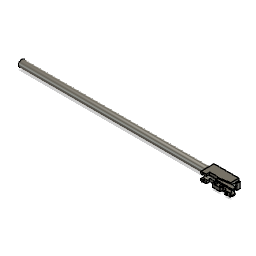
LP-point V2 (Autodesk Fusion 360 archive; units mm, degrees)
design "hp-995 barrel"
Autodesk Fusion 360 part; units mm, degrees
sketch "Sketch1" plane through (0, 0, 0) normal (0, 1, 0) x (1, 0, 0)
  line L0 (0, 0) -> (59, -0.000123)
  line L1 (0, 0) -> (59, -0.000123)
  line L2 (59, -0.000123) -> (58.999962, -18.000123)
  line L3 (0, 0) -> (-0.000063, -30)
  line L4 (-0.000063, -30) -> (4.999937, -30.00001)
  line L5 (4.999937, -30.00001) -> (4.999937, -29.00001)
  line L6 (4.999937, -29.000011) -> (11.499972, -29.000024)
  line L7 (11.499972, -29.000024) -> (11.499989, -21.000024)
  line L8 (11.499989, -21.000024) -> (30.499989, -21.000064)
  line L9 (30.49999, -21.000064) -> (30.499961, -34.49993)
  line L10 (59, -0.000123) -> (59, -11)
  line L11 (59, -0.000123) -> (58.999962, -18.000123)
  line L12 (58.999962, -18.000123) -> (64.000056, -18.000122)
  line L13 (68.499973, -21.000073) -> (68.499955, -30.000009)
  line L14 (68.499973, -21.000073) -> (64.000056, -18.000122)
  line L15 (68.499973, -21.000073) -> (68.499964, -25.500073)
  line L16 (70.000004, -33.000003) -> (70.000008, -31.000046)
  line L17 (0, 0) -> (59, -0.000123)
  line L18 (70.000008, -31.000046) -> (70.000004, -33.000003)
  line L19 (68.499955, -30.000009) -> (70.000008, -31.000046)
  line L20 (69.499995, -33.500012) -> (70.000004, -33.000003)
  line L21 (70, -35.000046) -> (70.000001, -34.5)
  circle A0 centre (34.5, -29.5) radius 2.5
  circle A1 centre (45.5, -29.5) radius 2.5
  line L22 (30.499961, -34.49993) -> (47.998896, -34.499967)
  line L23 (58.998896, -34.49999) -> (63.932836, -34.5)
  line L24 (50.387631, -29.964548) -> (56.610162, -29.964548)
  arc A2 (58.998896, -34.49999) -> (56.610162, -29.964548) centre (53.498896, -34.499967) ccw
  arc A3 (50.387631, -29.964548) -> (47.998896, -34.499967) centre (53.498896, -34.499967) ccw
  line L25 (63.932836, -34.5) -> (63.932838, -33.5)
  line L26 (63.932838, -33.5) -> (69.499995, -33.500012)
  dimension "d3" = 59
  dimension "d7" = 30
  dimension "d8" = 5
  dimension "d9" = 1
  dimension "d11" = 8
  dimension "d12" = 19
  dimension "d19" = 18
  dimension "d24" = 4.5
  dimension "d27" = 4
  dimension "d34" = 5.5
  dimension "d36" = 1
  constraint coincident L0.start L1.start
  constraint perpendicular L0 L2
  constraint perpendicular L1 L3
  constraint perpendicular L3 L4
  constraint vertical L5
  constraint perpendicular L3 L6
  constraint perpendicular L6 L7
  constraint perpendicular L7 L8
  constraint perpendicular L1 L9
  constraint perpendicular L0 L11
  constraint perpendicular L9 L22
  constraint parallel L13 L15
  constraint perpendicular L3 L17
  constraint perpendicular L17 L18
  constraint parallel L3 L13
  constraint collinear L22 L23
  constraint horizontal L24
  constraint concentric A2 A3
  constraint perpendicular L23 L25
  constraint perpendicular L25 L26
extrude "Extrude1" add sketch "Sketch1" along normal blind 18.5 contours L0 L1 L2 L3 L4 L5 L6 L7 L8 L9 L10 L11 L12 L13 L14 L15 L16 L17 L18 L19 L20 L22 L23 L24 A2 A3 L25 L26 picked at (29.83333, -7.000062) makes body 1
sketch "Sketch2" plane through (0, 0, 0) normal (1, 0, 0) x (0, 0, -1)
  line L0 (0, 0) -> (0, 18.5)
  line L1 (-19, 9.25) -> (-19, 9.252074)
  circle A0 centre (-11.4, 9.25) radius 7.6
  dimension "d39" = 18.5
  constraint coincident L0.start origin
  constraint vertical L0
  measures "d39" distance of L0.start L0.end
extrude "Extrude2" add sketch "Sketch2" against normal blind 422 contours L1 A0 picked at (-8.894962, 8.872426) bodies 1
sketch "Sketch3" plane through (0, 0, 0) normal (0, 1, 0) x (1, 0, 0)
sketch "Sketch4" plane through (0, 18.5, 0) normal (0, 1, 0) x (-1, 0, 0)
  circle A0 centre (-34.5, 29.5) radius 2.5
  circle A1 centre (-45.5, 29.5) radius 2.5
  line L0 (-58.998896, 34.49999) -> (-63.932836, 34.5)
  line L1 (-63.932836, 34.5) -> (-63.932838, 33.5)
  line L2 (-63.932838, 33.5) -> (-69.499995, 33.500012)
  line L3 (-69.499995, 33.500012) -> (-70.000004, 33.000003)
  line L4 (-70.000004, 33.000003) -> (-70.000008, 31.000046)
  line L5 (-70.000008, 31.000046) -> (-68.499955, 30.000009)
  line L6 (-68.499955, 30.000009) -> (-68.499973, 21.000073)
  line L7 (-68.499973, 21.000073) -> (-64.000056, 18.000122)
  line L8 (-64.000056, 18.000122) -> (-58.999962, 18.000123)
  line L9 (-58.999962, 18.000123) -> (-59, 0.000123)
  line L10 (-59, 0.000123) -> (0, 0)
  line L11 (0, 0) -> (0.000063, 30)
  line L12 (0.000063, 30) -> (-4.999937, 30.00001)
  line L13 (-4.999937, 30.00001) -> (-4.999937, 29.000011)
  line L14 (-4.999937, 29.000011) -> (-11.499972, 29.000024)
  line L15 (-11.499972, 29.000024) -> (-11.499989, 21.000024)
  line L16 (-11.499989, 21.000024) -> (-30.49999, 21.000064)
  line L17 (-30.49999, 21.000064) -> (-30.499961, 34.49993)
  line L18 (-30.499961, 34.49993) -> (-47.998896, 34.499967)
  arc A2 (-50.387631, 29.964548) -> (-47.998896, 34.499967) centre (-53.498896, 34.499967) ccw
  line L19 (-50.387631, 29.964548) -> (-56.610162, 29.964548)
  arc A3 (-58.998896, 34.49999) -> (-56.610162, 29.964548) centre (-53.498896, 34.499967) ccw
  line L20 (-58.999962, 18.000123) -> (-55.999962, 18.000117)
  line L21 (-55.999962, 18.000117) -> (-56, 0.000117)
  line L22 (-58.999962, 18.000123) -> (-59, 0.000123)
  line L23 (-59, 0.000123) -> (-56, 0.000117)
  dimension "d44" = 3
  constraint perpendicular L9 L20
  constraint perpendicular L10 L21
extrude "Extrude3" cut sketch "Sketch4" against normal blind 5 contours L9 L10 L20 L21 L22 L23 picked at (-57.999987, 6.000121) bodies 1
sketch "Sketch5" plane through (-422, 0, 0) normal (-1, 0, 0) x (0, 0, 1)
  circle A0 centre (11.4, 9.25) radius 7.6
  circle A1 centre (11.4, 9.25) radius 4.5
  dimension "d47" = 9
  constraint concentric A0 A1
  measures "d47" diameter of A1
extrude "Extrude4" cut sketch "Sketch5" against normal blind 500 contours A1 picked at (10.485657, 10.143968) bodies 1
sketch "Sketch6" plane through (0, 0, 0) normal (-1, 0, -0.00000209) x (-0.00000209, 0, 1)
  ellipse E0 centre (11.4, 9.25) end of major axis (3.8, 9.25) minor radius 7.6
  line L0 (0, 0) -> (30, 0)
  line L1 (30, 0) -> (30, 18.5)
  line L2 (30, 18.5) -> (0, 18.5)
  line L3 (0, 18.5) -> (0, 0)
  line L4 (30, 18.5) -> (30, 0)
  line L5 (25.100054, 14.248999) -> (30, 14.150928)
  line L6 (25.100054, 4.251001) -> (30, 4.349072)
  arc A0 (25.100054, 14.248999) -> (25.100054, 4.251001) centre (25, 9.25) ccw
  constraint coincident L1.end L2.start
  constraint coincident L0 L1.start
  constraint coincident L1 L0.end
  constraint tangent L5 A0
  constraint tangent L6 A0
extrude "Extrude5" cut sketch "Sketch6" against normal blind 29 contours L1 L4 L5 L6 A0 picked at (26.733369, 10.883643) bodies 1
sketch "Sketch7" plane through (0, 18.5, 0) normal (0, 1, 0) x (-1, 0, 0)
  line L0 (-55.999962, 18.000117) -> (-56, 0.000117)
  line L1 (-56, 0.000117) -> (0, 0)
  line L2 (0, 0) -> (0.000063, 30)
  line L3 (0.000063, 30) -> (-4.999937, 30.00001)
  line L4 (-4.999937, 30.00001) -> (-4.999937, 29.000011)
  line L5 (-4.999937, 29.000011) -> (-11.499972, 29.000024)
  line L6 (-11.499972, 29.000024) -> (-11.499989, 21.000024)
  line L7 (-11.499989, 21.000024) -> (-30.49999, 21.000064)
  line L8 (-30.49999, 21.000064) -> (-30.499961, 34.49993)
  line L9 (-30.499961, 34.49993) -> (-47.998896, 34.499967)
  arc A0 (-50.387631, 29.964548) -> (-47.998896, 34.499967) centre (-53.498896, 34.499967) ccw
  line L10 (-50.387631, 29.964548) -> (-56.610162, 29.964548)
  arc A1 (-58.998896, 34.49999) -> (-56.610162, 29.964548) centre (-53.498896, 34.499967) ccw
  line L11 (-58.998896, 34.49999) -> (-63.932836, 34.5)
  line L12 (-63.932836, 34.5) -> (-63.932838, 33.5)
  line L13 (-63.932838, 33.5) -> (-69.499995, 33.500012)
  line L14 (-69.499995, 33.500012) -> (-70.000004, 33.000003)
  line L15 (-70.000004, 33.000003) -> (-70.000008, 31.000046)
  line L16 (-70.000008, 31.000046) -> (-68.499955, 30.000009)
  line L17 (-68.499955, 30.000009) -> (-68.499973, 21.000073)
  line L18 (-68.499973, 21.000073) -> (-64.000056, 18.000122)
  line L19 (-64.000056, 18.000122) -> (-58.999962, 18.000123)
  line L20 (-58.999962, 18.000123) -> (-55.999962, 18.000117)
  circle A2 centre (-34.5, 29.5) radius 2.5
  circle A3 centre (-45.5, 29.5) radius 2.5
  line L21 (-30.499961, 34.49993) -> (-30.499978, 26.49993)
  line L22 (-30.499978, 26.49993) -> (-68.499962, 26.50001)
  dimension "d53" = 8
  constraint perpendicular L9 L21
  constraint perpendicular L17 L22
extrude "Extrude6" cut sketch "Sketch7" against normal blind 5.5 contours L8 L9 A0 L10 A1 L11 L12 L13 L14 L15 L16 L17 L21 L22 picked at (-63.388235, 30.329444) bodies 1
sketch "Sketch8" plane through (0, 0, 0) normal (0, -1, 0) x (1, 0, 0)
  circle A0 centre (34.5, 29.5) radius 2.5
  circle A1 centre (45.5, 29.5) radius 2.5
  line L0 (63.932836, 34.5) -> (58.998896, 34.49999)
  arc A2 (56.610162, 29.964548) -> (58.998896, 34.49999) centre (53.498896, 34.499967) ccw
  line L1 (56.610162, 29.964548) -> (50.387631, 29.964548)
  arc A3 (47.998896, 34.499967) -> (50.387631, 29.964548) centre (53.498896, 34.499967) ccw
  line L2 (47.998896, 34.499967) -> (30.499961, 34.49993)
  line L3 (30.499961, 34.49993) -> (30.49999, 21.000064)
  line L4 (30.49999, 21.000064) -> (11.499989, 21.000024)
  line L5 (11.499989, 21.000024) -> (11.499972, 29.000024)
  line L6 (11.499972, 29.000024) -> (4.999937, 29.000011)
  line L7 (4.999937, 29.000011) -> (4.999937, 30.00001)
  line L8 (4.999937, 30.00001) -> (-0.000063, 30)
  line L9 (-0.000063, 30) -> (0, 0)
  line L10 (0, 0) -> (59, 0.000123)
  line L11 (59, 0.000123) -> (58.999962, 18.000123)
  line L12 (58.999962, 18.000123) -> (64.000056, 18.000122)
  line L13 (64.000056, 18.000122) -> (68.499973, 21.000073)
  line L14 (68.499973, 21.000073) -> (68.499955, 30.000009)
  line L15 (68.499955, 30.000009) -> (70.000008, 31.000046)
  line L16 (70.000008, 31.000046) -> (70.000004, 33.000003)
  line L17 (70.000004, 33.000003) -> (69.499995, 33.500012)
  line L18 (69.499995, 33.500012) -> (63.932838, 33.5)
  line L19 (63.932838, 33.5) -> (63.932836, 34.5)
  line L20 (30.499961, 34.49993) -> (30.499978, 26.49993)
  line L21 (30.499978, 26.49993) -> (68.499962, 26.50001)
  dimension "d56" = 8
  constraint perpendicular L2 L20
  constraint perpendicular L14 L21
extrude "Extrude7" cut sketch "Sketch8" against normal blind 5.5 contours L0 A2 L1 A3 L2 L3 L14 L15 L16 L17 L18 L19 L20 L21 picked at (63.388235, 30.329444) bodies 1
sketch "Sketch9" plane through (0, 0, 0) normal (0, -1, 0) x (1, 0, 0)
  line L0 (68.499962, 26.50001) -> (30.499978, 26.49993)
  line L1 (30.499978, 26.49993) -> (30.49999, 21.000064)
  line L2 (30.49999, 21.000064) -> (11.499989, 21.000024)
  line L3 (11.499989, 21.000024) -> (11.499972, 29.000024)
  line L4 (11.499972, 29.000024) -> (4.999937, 29.000011)
  line L5 (4.999937, 29.000011) -> (4.999937, 30.00001)
  line L6 (4.999937, 30.00001) -> (-0.000063, 30)
  line L7 (-0.000063, 30) -> (0, 0)
  line L8 (0, 0) -> (59, 0.000123)
  line L9 (59, 0.000123) -> (58.999962, 18.000123)
  line L10 (58.999962, 18.000123) -> (64.000056, 18.000122)
  line L11 (64.000056, 18.000122) -> (68.499973, 21.000073)
  line L12 (68.499973, 21.000073) -> (68.499962, 26.50001)
  line L13 (30.499978, 26.49993) -> (30.499986, 22.49993)
  line L14 (30.499986, 22.49993) -> (68.49997, 22.50001)
  dimension "d59" = 4
  constraint perpendicular L0 L13
  constraint perpendicular L12 L14
extrude "Extrude8" cut sketch "Sketch9" against normal blind 2.5 contours L0 L1 L12 L13 L14 picked at (43.166642, 25.166623) bodies 1
sketch "Sketch10" plane through (0, 18.5, 0) normal (0, 1, 0) x (-1, 0, 0)
  line L0 (-30.499978, 26.49993) -> (-68.499962, 26.50001)
  line L1 (-68.499962, 26.50001) -> (-68.499973, 21.000073)
  line L2 (-68.499973, 21.000073) -> (-64.000056, 18.000122)
  line L3 (-64.000056, 18.000122) -> (-58.999962, 18.000123)
  line L4 (-58.999962, 18.000123) -> (-55.999962, 18.000117)
  line L5 (-55.999962, 18.000117) -> (-56, 0.000117)
  line L6 (-56, 0.000117) -> (0, 0)
  line L7 (0, 0) -> (0.000063, 30)
  line L8 (0.000063, 30) -> (-4.999937, 30.00001)
  line L9 (-4.999937, 30.00001) -> (-4.999937, 29.000011)
  line L10 (-4.999937, 29.000011) -> (-11.499972, 29.000024)
  line L11 (-11.499972, 29.000024) -> (-11.499989, 21.000024)
  line L12 (-11.499989, 21.000024) -> (-30.49999, 21.000064)
  line L13 (-30.49999, 21.000064) -> (-30.499978, 26.49993)
  line L14 (-30.499978, 26.49993) -> (-30.499986, 22.49993)
  line L15 (-30.499986, 22.49993) -> (-68.49997, 22.50001)
  dimension "d62" = 4
  constraint perpendicular L12 L14
  constraint perpendicular L1 L15
extrude "Extrude9" cut sketch "Sketch10" against normal blind 2.5 contours L0 L1 L13 L14 L15 picked at (-43.166642, 25.166623) bodies 1
sketch "Sketch11" plane through (0, 18.5, 0) normal (0, 1, 0) x (-1, 0, 0)
  line L0 (-30.499986, 22.49993) -> (-68.49997, 22.50001)
  line L1 (-68.49997, 22.50001) -> (-68.499973, 21.000073)
  line L2 (-68.499973, 21.000073) -> (-64.000056, 18.000122)
  line L3 (-64.000056, 18.000122) -> (-58.999962, 18.000123)
  line L4 (-58.999962, 18.000123) -> (-55.999962, 18.000117)
  line L5 (-55.999962, 18.000117) -> (-56, 0.000117)
  line L6 (-56, 0.000117) -> (0, 0)
  line L7 (0, 0) -> (0.000063, 30)
  line L8 (0.000063, 30) -> (-4.999937, 30.00001)
  line L9 (-4.999937, 30.00001) -> (-4.999937, 29.000011)
  line L10 (-4.999937, 29.000011) -> (-11.499972, 29.000024)
  line L11 (-11.499972, 29.000024) -> (-11.499989, 21.000024)
  line L12 (-11.499989, 21.000024) -> (-30.49999, 21.000064)
  line L13 (-30.49999, 21.000064) -> (-30.499986, 22.49993)
  line L14 (-30.499986, 22.49993) -> (-55.999962, 18.000117)
extrude "Extrude10" cut sketch "Sketch11" against normal blind 2.5 contours L0 L1 L2 L3 L4 L14 picked at (-51.66664, 21.000019) bodies 1
sketch "Sketch12" plane through (0, 0, 0) normal (0, -1, 0) x (1, 0, 0)
  line L0 (68.49997, 22.50001) -> (30.499986, 22.49993)
  line L1 (30.499986, 22.49993) -> (30.49999, 21.000064)
  line L2 (30.49999, 21.000064) -> (11.499989, 21.000024)
  line L3 (11.499989, 21.000024) -> (11.499972, 29.000024)
  line L4 (11.499972, 29.000024) -> (4.999937, 29.000011)
  line L5 (4.999937, 29.000011) -> (4.999937, 30.00001)
  line L6 (4.999937, 30.00001) -> (-0.000063, 30)
  line L7 (-0.000063, 30) -> (0, 0)
  line L8 (0, 0) -> (59, 0.000123)
  line L9 (59, 0.000123) -> (58.999962, 18.000123)
  line L10 (58.999962, 18.000123) -> (64.000056, 18.000122)
  line L11 (64.000056, 18.000122) -> (68.499973, 21.000073)
  line L12 (68.499973, 21.000073) -> (68.49997, 22.50001)
  line L13 (58.999962, 18.000123) -> (30.499986, 22.49993)
extrude "Extrude11" cut sketch "Sketch12" against normal blind 2.5 contours L0 L10 L11 L12 L13 picked at (52.66664, 21.000021) bodies 1
sketch "Sketch13" plane through (-0.000072, 0, 34.499867) normal (-0.00000209, 0, 1) x (1, 0, 0.00000209)
  line L0 (58.998968, 5.5) -> (63.932908, 5.5)
  line L1 (63.932908, 5.5) -> (63.932908, 13)
  line L2 (63.932908, 13) -> (58.998968, 13)
  line L3 (58.998968, 13) -> (58.998968, 5.5)
  circle A0 centre (61.465938, 9.25) radius 1.5
  dimension "d69" = 3
  measures "d69" diameter of A0
extrude "Extrude12" add sketch "Sketch13" along normal blind 1 contours A0 picked at (61.81025, 9.442709) bodies 1
sketch "Sketch14" plane through (0, 0, 0) normal (0, -1, 0) x (1, 0, 0)
  line L0 (58.999962, 18.000123) -> (30.499986, 22.49993)
  line L1 (30.499986, 22.49993) -> (30.49999, 21.000064)
  line L2 (30.49999, 21.000064) -> (11.499989, 21.000024)
  line L3 (11.499989, 21.000024) -> (11.499972, 29.000024)
  line L4 (11.499972, 29.000024) -> (4.999937, 29.000011)
  line L5 (4.999937, 29.000011) -> (4.999937, 30.00001)
  line L6 (4.999937, 30.00001) -> (-0.000063, 30)
  line L7 (-0.000063, 30) -> (0, 0)
  line L8 (0, 0) -> (59, 0.000123)
  line L9 (59, 0.000123) -> (58.999962, 18.000123)
  line L10 (59, 0.000123) -> (58.999984, 7.500123)
  line L11 (58.999984, 7.500123) -> (55.999984, 7.500117)
  line L12 (55.999972, 13.500117) -> (58.999972, 13.500123)
  line L13 (58.999984, 7.500123) -> (55.999984, 7.500117)
  line L14 (55.999984, 7.500117) -> (55.999972, 13.500117)
  dimension "d72" = 7.5
  dimension "d75" = 3
  constraint perpendicular L8 L10
  constraint perpendicular L9 L11
  constraint perpendicular L9 L12
  constraint perpendicular L9 L13
  constraint perpendicular L12 L14
extrude "Extrude13" cut sketch "Sketch14" against normal blind 20 contours L9 L11 L12 L13 L14 picked at (56.99998, 9.500119) bodies 1
sketch "Sketch15" plane through (59, 0, 0.000123) normal (1, 0, 0.00000209) x (0.00000209, 0, -1)
  line L0 (-13.5, 0) -> (-13.5, 5.270115)
  arc A0 (-13.5, 13.229885) -> (-13.5, 5.270115) centre (-11.399877, 9.25) ccw
  line L1 (-13.5, 13.229885) -> (-13.5, 13.5)
  line L2 (-13.5, 13.5) -> (-18, 13.5)
  line L3 (-18, 13.5) -> (-18, 2.5)
  line L4 (-18, 2.5) -> (-18, 0)
  line L5 (-18, 0) -> (-13.5, 0)
sketch "Sketch16" plane through (51.500017, 0, 51.499997) normal (0.70710691, 0, 0.70710665) x (0.70710665, 0, -0.70710691)
  line L0 (25.455819, 5.5) -> (26.162938, 5.5)
  line L1 (26.162938, 5.5) -> (26.162938, 13)
  line L2 (26.162938, 13) -> (25.455819, 13)
  line L3 (25.455819, 13) -> (25.455819, 5.5)
  line L4 (25.455819, 9.25) -> (26.162938, 9.25)
  line L5 (26.162938, 9.25) -> (30.662938, 9.25)
  circle A0 centre (30.662938, 9.25) radius 4.5
  dimension "d79" = 9
  constraint perpendicular L1 L5
  measures "d79" diameter of A0
extrude "Extrude14" cut sketch "Sketch16" against normal blind 25 contours A0 picked at (32.430079, 10.270259) bodies 1 makes body 2 at (58.974168, 13.499091, 13.51487)

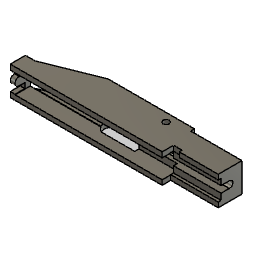
design "995 bolt"
Autodesk Fusion 360 part; units mm, degrees
sketch "Sketch1" plane through (0, 0, 0) normal (0, 1, 0) x (1, 0, 0)
  line L0 (65, 0) -> (156, 0)
  line L1 (0, -22) -> (0, -38)
  line L2 (210, -4) -> (210, -29)
  line L3 (160, -38) -> (0, -38)
  line L4 (156, 0) -> (156, -4)
  line L5 (156, -4) -> (210, -4)
  line L6 (0, -38) -> (0, -22)
  line L7 (0, -22) -> (10, -22)
  line L8 (10, -22) -> (65, 0)
  line L9 (210, 0) -> (135, 0)
  circle A0 centre (135, -8.75) radius 3.25
  line L10 (160, -38) -> (160, -29)
  line L11 (160, -29) -> (210, -29)
  dimension "d2" = 38
  dimension "d5" = 4
  dimension "d6" = 16
  dimension "d7" = 10
  dimension "d8" = 65
  dimension "d9" = 75
  dimension "d13" = 9
  constraint horizontal L0
  constraint perpendicular L0 L1
  constraint perpendicular L0 L2
  constraint perpendicular L0 L4
  constraint perpendicular L4 L5
  constraint perpendicular L3 L6
  constraint perpendicular L1 L7
  constraint parallel L0 L9
  constraint perpendicular L3 L10
  constraint perpendicular L10 L11
  measures "d2" distance of origin L1.end
  measures "d5" distance of L0.end L4.end
  measures "d6" distance of L1.end L1.start
  measures "d7" distance of L1.start L7.end
  measures "d8" distance of origin L0.start
  measures "d9" distance of L9.start L9.end
  measures "d13" distance of L3.start L10.end
extrude "Extrude1" add sketch "Sketch1" along normal blind 30.5
sketch "Sketch2" plane through (0, 30.5, 0) normal (0, 1, 0) x (-1, 0, 0)
  circle A0 centre (-135, 8.75) radius 3.25
  line L0 (-160, 38) -> (-160, 29)
  line L1 (-160, 29) -> (-210, 29)
  line L2 (-210, 29) -> (-210, 4)
  line L3 (-210, 4) -> (-156, 4)
  line L4 (-156, 4) -> (-156, 0)
  line L5 (-156, 0) -> (-65, 0)
  line L6 (-65, 0) -> (-10, 22)
  line L7 (-10, 22) -> (0, 22)
  line L8 (0, 22) -> (0, 38)
  line L9 (0, 38) -> (-160, 38)
  line L10 (-160, 29) -> (-160, 26)
  line L11 (-160, 26) -> (-169, 26)
  line L12 (-169, 26) -> (-169, 29)
  dimension "d16" = 3
  dimension "d17" = 9
  constraint coincident L0.end L1.start
  constraint perpendicular L1 L10
  constraint perpendicular L10 L11
  constraint coincident L1 L12.end
  constraint perpendicular L1 L12
  measures "d16" distance of L0.end L10.end
  measures "d17" distance of L10.end L11.end
extrude "Extrude2" cut sketch "Sketch2" against normal blind 5.5 contours L1 L10 L11 L12
sketch "Sketch3" plane through (0, 0, 0) normal (-1, 0, 0) x (0, 0, 1)
  line L0 (22, 0) -> (38, 0)
  line L1 (38, 0) -> (38, 30.5)
  line L2 (38, 30.5) -> (22, 30.5)
  line L3 (22, 30.5) -> (22, 0)
  line L4 (22, 15.25) -> (38, 15.25)
  line L5 (38, 15.25) -> (33.75, 15.25)
  line L6 (22, 30.5) -> (27.5, 30.5)
  line L7 (33.75, 11) -> (27.5, 11)
  line L8 (33.9717, 19.4942) -> (27.5, 19.4942)
  arc A0 (33.75, 11) -> (33.5283, 19.4942) centre (33.75, 15.25) ccw
  line L9 (27.5, 30.5) -> (27.5, 19.4942)
  line L10 (27.5, 11) -> (27.5, 0)
  line L11 (33.9717, 24.9942) -> (27.5, 24.9942)
  line L12 (33.75, 5.5) -> (27.5, 5.5)
  line L13 (33.75, 5.5) -> (38, 5.5)
  line L14 (33.9717, 24.9942) -> (38, 24.9942)
  dimension "d20" = 4.25
  dimension "d21" = 5.5
  dimension "d22" = 5.5
  dimension "d23" = -5.5
  constraint midpoint L3 L4.start
  constraint midpoint L1 L4.end
  constraint parallel L4 L5
  constraint coincident L5.end A0.centre
  constraint coincident L4.end A0
  constraint coincident L2.end L3.start
  constraint perpendicular L3 L6
  constraint perpendicular L6 L9
  constraint coincident L7.end L9
  constraint tangent L7 A0
  constraint perpendicular L7 L9
  constraint coincident L8.start A0
  constraint perpendicular L8 L9
  constraint coincident L8 A0.end
  constraint collinear L9 L10
  constraint coincident L1 L13.end
  constraint perpendicular L1 L13
  constraint coincident L1 L14.end
  constraint perpendicular L1 L14
  measures "d20" distance of L4.end L5.end
  measures "d21" distance of L2.end L6.end
extrude "Extrude3" cut sketch "Sketch3" against normal blind 300 contours L1 L7 A0 L10 L12 L13 | L1 L8 A0 L9 L11 L14
sketch "Sketch4" plane through (0, 0, 38) normal (0, 0, 1) x (1, 0, 0)
  line L0 (0, 24.9942) -> (160, 24.9942)
  line L1 (160, 24.9942) -> (160, 30.5)
  line L2 (160, 30.5) -> (0, 30.5)
  line L3 (0, 30.5) -> (0, 24.9942)
  line L4 (0, 19) -> (0, 11)
  line L5 (0, 11) -> (5, 11)
  line L6 (5, 11) -> (5, 24.9942)
  line L7 (5, 24.9942) -> (5, 5)
  line L8 (160, 24.9942) -> (160, 5)
  line L9 (160, 5) -> (5, 5)
  line L10 (5, 5) -> (5, 27)
  line L11 (160, 24.9942) -> (5, 24.9942)
  dimension "d26" = 5
  dimension "d27" = 155
  constraint perpendicular L0 L4
  constraint perpendicular L3 L5
  constraint coincident L0 L6.end
  constraint perpendicular L0 L6
  constraint perpendicular L0 L7
  constraint coincident L0.end L1.start
  constraint perpendicular L0 L8
  constraint perpendicular L7 L9
  constraint perpendicular L0 L10
  constraint perpendicular L8 L11
  measures "d26" distance of L4.end L5.end
  measures "d27" distance of L0.end L6.end
extrude "Extrude4" cut sketch "Sketch4" against normal blind 16 contours L0 L6 L7 L8 L9 L10 L11
sketch "Sketch5" plane through (0, 0, 0) normal (-1, 0, 0) x (0, 0, 1)
  line L0 (38, 5.5) -> (27.5, 5.5)
  line L1 (27.5, 5.5) -> (27.5, 11)
  line L2 (27.5, 11) -> (33.75, 11)
  arc A0 (33.75, 11) -> (33.5283, 19.4942) centre (33.75, 15.25) ccw
  line L3 (33.5283, 19.4942) -> (27.5, 19.4942)
  line L4 (27.5, 19.4942) -> (27.5, 24.9942)
  line L5 (27.5, 24.9942) -> (38, 24.9942)
  line L6 (38, 24.9942) -> (38, 30.5)
  line L7 (38, 30.5) -> (22, 30.5)
  line L8 (22, 30.5) -> (22, 0)
  line L9 (22, 0) -> (38, 0)
  line L10 (38, 0) -> (38, 5.5)
  line L11 (27.5, 19.4942) -> (27.5, 11)
  line L12 (25.5, 19.4942) -> (25.5, 11)
  line L13 (25.5, 15.2471) -> (18.5, 15.2471)
  circle A1 centre (18.5, 15.2471) radius 7
  dimension "d33" = 2
  dimension "d34" = 7
  dimension "d35" = 14
  constraint coincident L3.end L4.start
  constraint coincident L1.end L2.start
  constraint midpoint L12 L13.start
  constraint perpendicular L8 L13
  constraint coincident L13.end A1.centre
  measures "d34" distance of L13.start L13.end
  measures "d35" diameter of A1
extrude "Extrude5" cut sketch "Sketch5" against normal blind 5 contours L8 A1 | L8 L13 A1 | L8 L13 A1
sketch "Sketch6" plane through (0, 0, 0) normal (-1, 0, 0) x (0, 0, 1)
  arc A0 (22, 9.1849) -> (22, 21.3093) centre (18.5, 15.2471) ccw
  line L0 (22, 9.1849) -> (22, 0)
  line L1 (22, 0) -> (38, 0)
  line L2 (38, 0) -> (38, 5.5)
  line L3 (38, 5.5) -> (27.5, 5.5)
  line L4 (27.5, 5.5) -> (27.5, 11)
  line L5 (27.5, 11) -> (33.75, 11)
  arc A1 (33.75, 11) -> (33.5283, 19.4942) centre (33.75, 15.25) ccw
  line L6 (33.5283, 19.4942) -> (27.5, 19.4942)
  line L7 (27.5, 19.4942) -> (27.5, 24.9942)
  line L8 (27.5, 24.9942) -> (38, 24.9942)
  line L9 (38, 24.9942) -> (38, 30.5)
  line L10 (38, 30.5) -> (22, 30.5)
  line L11 (22, 30.5) -> (22, 21.3093)
  line L12 (22, 30.5) -> (0, 30.5)
  line L13 (22, 25) -> (5.5, 25)
  line L14 (0, 0) -> (22, 0)
  line L15 (5.5, 5.5) -> (22, 5.5)
  line L16 (5.5, 5.5) -> (5.5, 25)
  constraint coincident L10.end L11.start
  constraint perpendicular L11 L12
  constraint coincident L14.start origin
  constraint coincident L0.end L1.start
  constraint perpendicular L13 L16
  constraint parallel L12 L13
  constraint parallel L14 L15
extrude "Extrude6" cut sketch "Sketch6" against normal blind 114 contours A0 L0 L11 L13 L15 L16
sketch "Sketch7" plane through (210, 0, 0) normal (1, 0, 0) x (0, 0, -1)
  line L0 (-29, 11) -> (-27.5, 11)
  line L1 (-27.5, 11) -> (-27.5, 5.5)
  line L2 (-27.5, 5.5) -> (-29, 5.5)
  line L3 (-29, 5.5) -> (-29, 0)
  line L4 (-29, 0) -> (-4, 0)
  line L5 (-4, 0) -> (-4, 30.5)
  line L6 (-4, 30.5) -> (-29, 30.5)
  line L7 (-29, 30.5) -> (-29, 24.9942)
  line L8 (-29, 24.9942) -> (-27.5, 24.9942)
  line L9 (-27.5, 24.9942) -> (-27.5, 19.4942)
  line L10 (-27.5, 19.4942) -> (-29, 19.4942)
  line L11 (-29, 19.4942) -> (-29, 11)
  circle A0 centre (-17, 15.25) radius 3.5
  line L12 (-29, 25.3) -> (-26, 25.3)
  line L13 (-29, 5.2) -> (-26, 5.2)
  line L14 (-17, 15.25) -> (-17, 18.75)
  line L15 (-17, 18.75) -> (-26, 18.75)
  line L16 (-17.3755, 11.7702) -> (-26, 11.7702)
  line L17 (-26, 25.3) -> (-26, 18.75)
  line L18 (-26, 11.7702) -> (-26, 5.2)
  line L19 (-29, 5.2) -> (-29, 25.3)
  dimension "d44" = 7
  dimension "d45" = 5.2
  dimension "d46" = 3
  dimension "d47" = 5.2
  dimension "d48" = 3
  constraint perpendicular L7 L12
  constraint perpendicular L1 L13
  constraint coincident A0.centre L14.start
  constraint coincident A0 L14.end
  constraint tangent A0 L15
  constraint coincident A0 L16.start
  constraint coincident L16.end L17
  constraint perpendicular L16 L17
  constraint collinear L17 L18
  measures "d44" diameter of A0
  measures "d45" distance of L6.end L12.start
  measures "d46" distance of L12.start L12.end
  measures "d47" distance of L3.end L13.start
  measures "d48" distance of L13.start L13.end
extrude "Extrude7" cut sketch "Sketch7" against normal blind 93.5 contours L0 L1 L2 L3 L7 L8 L9 L10 L11 A0 L12 L13 L15 L16 L17 L18 L19 | L0 L1 L2 L19 | L8 L9 L10 L19 | A0
sketch "Sketch8" plane through (0, 0, 0) normal (0, -1, 0) x (1, 0, 0)
  circle A0 centre (135, 8.75) radius 3.25
  line L0 (160, 29) -> (160, 38)
  line L1 (160, 38) -> (0, 38)
  line L2 (0, 38) -> (0, 22)
  line L3 (0, 22) -> (10, 22)
  line L4 (10, 22) -> (65, 0)
  line L5 (65, 0) -> (156, 0)
  line L6 (156, 0) -> (156, 4)
  line L7 (156, 4) -> (210, 4)
  line L8 (210, 4) -> (210, 29)
  line L9 (210, 29) -> (160, 29)
  line L10 (210, 16.5) -> (119.5, 16.5)
  line L11 (120, 8.5) -> (119.5, 26.5)
  line L12 (120, 8.5) -> (84.7086, 8.5)
  line L13 (119.5, 26.5) -> (84.7086, 26.5)
  arc A1 (84.7086, 26.5) -> (84.7086, 8.5) centre (87.75, 17.5) ccw
  dimension "d51" = 90.5
  dimension "d55" = 19
  constraint midpoint L8 L10.start
  constraint perpendicular L8 L10
  constraint parallel L12 L13
  measures "d51" distance of L10.start L10.end
  measures "d55" diameter of A1
extrude "Extrude8" cut sketch "Sketch8" against normal blind 25 contours L11 L12 L13 A1
